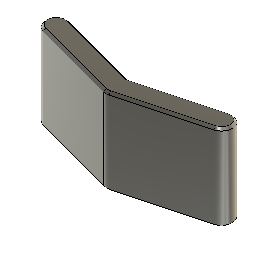
FRIDGEMAGswitch (Autodesk Fusion 360 design; units mm, degrees)
Autodesk Fusion 360 part; units mm, degrees
sketch "Sketch1" plane through (0, 0, 0) normal (0, 0, 1) x (1, 0, 0)
  line L0 (0, 0) -> (38.637, 10.3528) construction
  line L1 (0, 0) -> (39, 0) construction
  line L2 (0.647, -2.4148) -> (19.9656, 2.7616)
  arc A0 (19.9656, 2.7616) -> (18.6715, 7.5912) centre (19.3185, 5.1764) ccw
  line L3 (18.6715, 7.5912) -> (-0.647, 2.4148)
  arc A1 (-0.647, 2.4148) -> (0.647, -2.4148) centre (0, 0) ccw
  line L4 (0, 0) -> (19.3185, 5.1764) construction
  line L5 (0, 0) -> (0, 50) construction
  arc A2 (-18.6715, 7.5912) -> (-19.9656, 2.7616) centre (-19.3185, 5.1764) ccw
  line L6 (-18.6715, 7.5912) -> (0.647, 2.4148)
  line L7 (0, 0) -> (-19.3185, 5.1764) construction
  arc A3 (-0.647, -2.4148) -> (0.647, 2.4148) centre (0, 0) ccw
  line L8 (-0.647, -2.4148) -> (-19.9656, 2.7616)
  line L9 (1.673, 1.4836) -> (16.1619, 5.3658)
  line L10 (16.1619, 5.3658) -> (16.6796, 3.434)
  line L11 (16.6796, 3.434) -> (2.1907, -0.4483)
  line L12 (2.1907, -0.4483) -> (1.673, 1.4836)
  line L13 (-1.673, 1.4836) -> (-16.1619, 5.3658)
  line L14 (-16.6796, 3.434) -> (-2.1907, -0.4483)
  line L15 (-16.1619, 5.3658) -> (-16.6796, 3.434)
  line L16 (-2.1907, -0.4483) -> (-1.673, 1.4836)
  dimension "d6" = 40
  dimension "d7" = 15
  dimension "d8" = 5
  dimension "d12" = 20
  dimension "d13" = 50
  dimension "d15" = 15
  dimension "d16" = 2
  dimension "d17" = 2
  dimension "d18" = 1.5
  constraint horizontal L1
  constraint coincident L0.start L1.start
  constraint tangent L2 A0
  constraint tangent A0 L3
  constraint parallel L2 L3
  constraint tangent L3 A1
  constraint tangent L2 A1
  constraint parallel L0 L4
  constraint perpendicular L1 L5
  constraint symmetric L0.start L5 L1.start
  constraint symmetric L2.start L5 A3.start
  constraint symmetric L2.end L5 A2.end
  constraint symmetric A0.end L5 A2.start
  constraint symmetric L3.end L5 L6.end
  constraint symmetric A0 L5 A2
  constraint symmetric A1 L5 A3
  constraint perpendicular L9 L10
  constraint parallel L9 L11
  constraint parallel L10 L12
  constraint parallel L3 L9
  constraint symmetric L5 L9.start L13.start
  constraint symmetric L5 L9.end L13.end
  constraint symmetric L5 L10.end L14.start
  constraint symmetric L5 L11.end L14.end
  measures "d6" distance of L0.start L0.end
  measures "d7" angle of L0 L1
  measures "d8" diameter of A0
  measures "d12" distance of L0.start A0.centre
  measures "d13" distance of L0.start L5.end
  measures "d15" distance of L9.start L9.end
  measures "d16" distance of L9.end L10.end
  measures "d17" distance of L0.start L12
  measures "d18" distance of L2 L10.end
extrude "Extrude1" add sketch "Sketch1" along normal blind 20 in component "magbody"
extrude "Extrude2" cut sketch "Sketch1" along normal blind 15 from surface at 2.5 contours A3 L9 L11 L12 | A3 L9 L10 L11 | A1 L13 L14 L15 | A1 L13 L14 L16 in component "magbody"
chamfer "Chamfer1" distance 0.5 angle 45 7 edges at (10.3063, 0.1734, 20) (0, -2.5, 20) (-10.3063, 0.1734, 20) (-21.7333, 5.8234, 20) (-9.3357, 5.0897, 20) (9.3357, 5.0897, 20) (21.7333, 5.8234, 20) in component "magbody"
chamfer "Chamfer1" distance 0.5 angle 45 7 edges at (10.3063, 0.1734, 0) (21.7333, 5.8234, 0) (9.3357, 5.0897, 0) (-9.3357, 5.0897, 0) (-21.7333, 5.8234, 0) (-10.3063, 0.1734, 0) (0, -2.5, 0) in component "magbody"
component "magbody" placed x (1, 0, 0) y (0, 1, 0) z (0, 0, 1) at (0, 0, 0)
